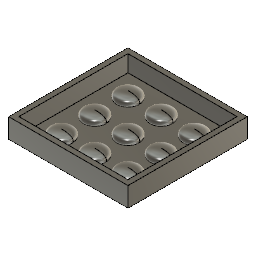
go_stones_mold (Autodesk Fusion 360 design; units mm, degrees)
Autodesk Fusion 360 part; units mm, degrees
sketch "Sketch1" plane through (0, 0, 0) normal (0, 1, 0) x (1, 0, 0)
  line L0 (0, 0) -> (0, -6.2)
  line L1 (0, 0) -> (10.7, 0)
  spline S0 degree 5 poles (10.7, 0) (10.7559, -0.0473) (10.8614, -0.1544) (11.0004, -0.3531) (11.1471, -0.6945) (11.2577, -1.2444) (11.2749, -1.8995) (11.1572, -2.6167) (10.8507, -3.3335) (10.3193, -3.992) (9.5498, -4.5477) (8.6121, -5.0047) (7.56, -5.3794) (6.3963, -5.6787) (5.1024, -5.9095) (3.6416, -6.0751) (2.3072, -6.1567) (1.1977, -6.1894) (0.4076, -6.1986) (0, -6.2) knots 0 0 0 0 0 0 0.066667 0.133333 0.2 0.266667 0.333333 0.4 0.466667 0.533333 0.6 0.666667 0.733333 0.8 0.866667 0.933333 1 1 1 1 1 1
  line L2 (2.4497, -6.1915) -> (-2.4497, -6.2085)
  line L3 (10.7986, -3.7001) -> (8.5, -5.171)
  point P0 (11.25, -1.5)
  point P1 (11.25, -1.5)
  point P2 (9.6493, -4.4355)
  dimension "d1" = 6.2
  dimension "d2" = 10.7
  dimension "d5" = 1.5
  dimension "d6" = 11.25
  constraint coincident L0.start L1.start
  constraint vertical L0
  constraint perpendicular L0 L1
  constraint coincident P1 P0
  constraint midpoint L0.end L2
  constraint midpoint P2 L3
  measures "d1" distance of L0.start L0.end
  measures "d2" distance of L0.start L1.end
  measures "d5" distance of L1 P1
  measures "d6" distance of L0 P1
revolve "Revolve1" add sketch "Sketch1" angle 360 about axis through (0, 0, 0) along (0, 0, 1) makes body 1
pattern_linear "R-Pattern1" count 3 spacing 32 along (0, 1, 0) count 3 spacing 32 along (-1, 0, 0) of bodies 1 makes body 2 at (6.1006, 26.3395, 0) makes body 3 at (7.4981, 67.6109, 0) makes body 4 at (-35.0404, -7.7469, 0) makes body 5 at (-35.0404, 24.2531, 0) makes body 6 at (-24.5019, 67.6109, 0) makes body 7 at (-69.1888, -6.5066, 0) makes body 8 at (-69.1888, 38.5066, 0) makes body 9 at (-56.5019, 67.6109, 0)
sketch "Sketch2" plane through (0, 0, 0) normal (0, 0, 1) x (1, 0, 0)
  line L0 (-85, -20) -> (20, -20)
  line L1 (20, -20) -> (20, 85)
  line L2 (20, 85) -> (-85, 85)
  line L3 (-85, 85) -> (-85, -20)
  line L4 (25, -25) -> (25, 90)
  line L5 (25, 90) -> (-90, 90)
  line L6 (-90, 90) -> (-90, -25)
  line L7 (-90, -25) -> (25, -25)
  dimension "d14" = 5
  constraint horizontal L0
  constraint vertical L1
  constraint horizontal L2
  constraint vertical L3
extrude "Extrude1" add sketch "Sketch2" along normal blind 16 and the other way blind 3 separate body makes body 10
extrude "Extrude2" add sketch "Sketch2" against normal blind 3 contours L0 L1 L2 L3 bodies 1 2 3 4 5 6 7 8 9 10
